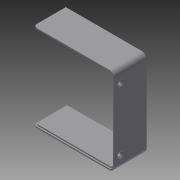
# Autodesk Inventor part: SimpleFrontLeftPlate
Saved by Autodesk Inventor 2015 (Build 190159000, 159)
## iProperties
Created: 2015-07-12
Part Number: SimpleFrontLeftPlate
Material: Generic
Document SubType Name: Modeling
Designer: -
Density: 1 g/cm^3
Appearance: Default
Author: -
Autodesk Inventor part; units mm, degrees
ref_plane "YZ Plane" through (0, 0, 0) normal (1, 0, 0) x (0, 1, 0)
ref_plane "XZ Plane" through (0, 0, 0) normal (0, 1, 0) x (-1, 0, 0)
ref_plane "XY Plane" through (0, 0, 0) normal (0, 0, 1) x (1, 0, 0)
ref_plane "Work Plane1" through (0, 0, 0) normal (0, 0, 1) x (1, 0, 0)
sketch "Sketch1" plane through (0, 0, 0) normal (0, 0, 1) x (1, 0, 0)
  line L0 (22.0847, -27.765) -> (20.0847, -27.765) projected
  line L1 (20.0847, -27.765) -> (20.0847, -26.575) projected
  arc A0 (16.0847, -30.575) -> (20.0847, -26.575) centre (16.0847, -26.575) ccw projected
  line L2 (16.0847, -30.575) -> (-40.4221, -30.575) projected
  line L3 (-40.4221, -30.575) -> (-40.4221, -34.575) projected
  line L4 (-40.4221, -34.575) -> (20.0847, -34.575) projected
  arc A1 (20.0847, -34.575) -> (24.0847, -30.575) centre (20.0847, -30.575) ccw projected
  line L5 (24.0847, -30.575) -> (24.0847, 30.575) projected
  arc A2 (24.0847, 30.575) -> (20.0847, 34.575) centre (20.0847, 30.575) ccw projected
  line L6 (20.0847, 34.575) -> (-40.4221, 34.575) projected
  line L7 (-40.4221, 34.575) -> (-40.4221, 30.575) projected
  line L8 (-40.4221, 30.575) -> (16.0847, 30.575) projected
  arc A3 (20.0847, 26.575) -> (16.0847, 30.575) centre (16.0847, 26.575) ccw projected
  line L9 (20.0847, 26.575) -> (20.0847, 27.765) projected
  line L10 (20.0847, 27.765) -> (22.0847, 27.765) projected
  line L11 (22.0847, 27.765) -> (22.0847, 21.765) projected
  line L12 (22.0847, 21.765) -> (20.0847, 21.765) projected
  line L13 (20.0847, 21.765) -> (20.0847, -21.765) projected
  line L14 (20.0847, -21.765) -> (22.0847, -21.765) projected
  line L15 (22.0847, -21.765) -> (22.0847, -27.765) projected
  line L16 (-40.4221, 34.575) -> (24.0847, 34.575)
  line L17 (24.0847, 34.575) -> (24.0847, -34.575)
  line L18 (24.0847, -34.575) -> (-40.4221, -34.575)
  line L19 (-40.4221, -32.575) -> (20.0847, -32.575)
  line L20 (22.0847, -30.575) -> (22.0847, 30.575)
  line L21 (20.0847, 32.575) -> (-40.4221, 32.575)
  arc A4 (22.0847, 30.575) -> (20.0847, 32.575) centre (20.0847, 30.575) ccw
  arc A5 (20.0847, -32.575) -> (22.0847, -30.575) centre (20.0847, -30.575) ccw
  point P0 (0, 0)
  dimension "d0" = 2
  dimension "d1" = 2
  dimension "d2" = 2
  constraints: 12 end point, 4 point on circle, 4 tangent, 2 centre point, 2 midpoint, 2 point on line, 1 collinear, 1 equal radius, 1 horizontal, 1 perpendicular
  measures "d0" distance between parallel lines of L6 L21
  measures "d1" distance between parallel lines of L20 L5
  measures "d2" radius of A4
extrude "Extrusion1" add sketch "Sketch1" along normal blind 25 contours L15 L20 L11 A4 L21 L7 L6 A2 L5 A1 L4 L3 L19 A5
sketch "Sketch2" plane through (24.0847, -30.575, 0) normal (1, 0, 0) x (0, 0, -1)
  circle A0 centre (-21.085, 55.34) radius 1.4 projected
  circle A1 centre (-21.085, 5.81) radius 1.4 projected
  point P0 (0, 30.575)
extrude "Extrusion2" cut sketch "Sketch2" against normal blind 25
chamfer "Chamfer1" distance 1 angle 45 2 edges at (24.0847, 24.765, 22.485) (24.0847, -24.765, 22.485)
lip "Lip1" kind lip height 1 width 1 edges at (-10.1687, 34.575, 25) (22.9131, 33.4034, 25) (24.0847, 0, 25) (22.9131, -33.4034, 25) (-10.1687, -34.575, 25) guide face at (22.7513, 10.1917, 25)
lip "Lip4" kind groove height 1 width 1 edges at (-40.4221, -32.575, 12.5) guide face at (-40.4221, -33.575, 8.3333)
lip "Lip5" kind groove height 1 width 1 edges at (-40.4221, 32.575, 12.5) guide face at (-40.4221, 33.575, 8.3333)
fillet "Fillet3" radius 3 2 edges at (-40.4221, -34.075, 26) (-40.4221, 34.075, 26)
fillet "Fillet4" radius 2 2 edges at (-39.4221, 33.075, 25) (-39.4221, -33.075, 25)
body "Solid1"
